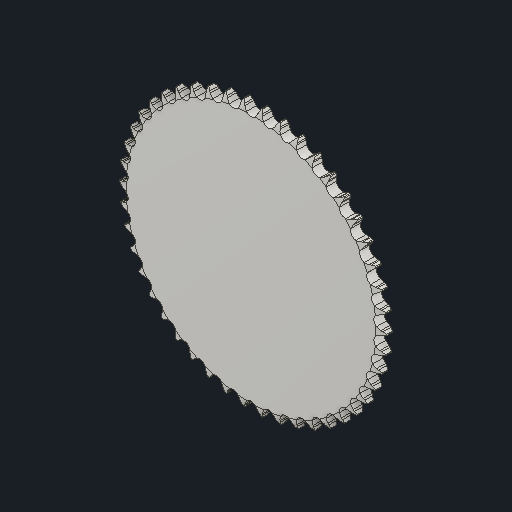
# Autodesk Inventor part: Roller Chain Sprocket2
Saved by Autodesk Inventor 2027 (Build 310192000, 192)
## iProperties
CustomPartVersion: 1
Created: 2026-06-06
Part Number: Roller Chain Sprocket2
Material: Steel
Document SubType Name: Modeling
Designer: W Ahmad
Density: 1 g/cm^3
Appearance: Steel
Author: W Ahmad
Autodesk Inventor part; units mm, degrees
ref_plane "YZ Plane" through (0, 0, 0) normal (1, 0, 0) x (0, 1, 0)
ref_plane "XZ Plane" through (0, 0, 0) normal (0, 1, 0) x (-1, 0, 0)
sketch "Theoretical Tooth Profile" plane through (0, 0, 0) normal (0, 0, 1) x (1, 0, 0)
  circle A0 centre (0, 0) radius 116.3133 construction
  line L0 (0, 0) -> (0, 116.3133) construction
  line L1 (0, 0) -> (15.838, 115.2299) construction
  circle A1 centre (0, 0) radius 120.8046
  arc A2 (-4.1451, 113.268) -> (4.1451, 113.268) centre (0, 116.3133) ccw
  line L2 (0, 116.3133) -> (15.838, 115.2299) construction
  line L3 (0, 116.3133) -> (6.5502, 121.1257) construction
  line L4 (6.5502, 121.1257) -> (-5.9584, 116.6908) construction
  arc A3 (7.8437, 120.5497) -> (6.453, 118.086) centre (14.1908, 115.3426) ccw
  arc A4 (-6.453, 118.086) -> (-7.8437, 120.5497) centre (-14.1908, 115.3426) ccw
  line L5 (-14.1908, 115.3426) -> (-6.453, 118.086) construction
  arc A5 (-5.9584, 116.6908) -> (-4.1451, 113.268) centre (6.5502, 121.1257) ccw
  line L6 (-5.9584, 116.6908) -> (-6.453, 118.086)
  arc A6 (4.1451, 113.268) -> (5.9584, 116.6908) centre (-6.5502, 121.1257) ccw
  line L7 (6.453, 118.086) -> (5.9584, 116.6908)
  line L8 (0, 0) -> (8.244, 120.523) construction
  point P0 (7.919, 115.7716)
  dimension "d0" = 232.6266
  dimension "d2" = 7.826
  dimension "d3" = 5.1435
  dimension "d10" = 126.304
  dimension "d11" = 16.783
  dimension "d12" = 8.128
  dimension "d13" = 13.2715
  dimension "d14" = 14.224
  dimension "d23" = 4.7625
  constraints: 18 end point, 15 point on circle, 7 centre point, 3 coincident, 3 point on line, 3 symmetric about line, 3 tangent, 1 equal radius, 1 midpoint, 1 parallel, 1 vertical, 1 other
  measures "d0" diameter of A0
  measures "d2" angle of L1 L0
  measures "d3" radius of A2
  measures "d10" angle of L3 L0
  measures "d11" angle of L4 L3
  measures "d12" distance of L2.start L3.end
  measures "d13" distance of L3.end L4.end
  measures "d14" distance of A3.centre L0.end
  measures "d23" distance from line of L8.end L2
sketch "Tooth Profile" plane through (0, 0, 0) normal (0, 0, 1) x (1, 0, 0)
  circle A0 centre (0, 0) radius 120.8046 projected
  line L0 (0, 0) -> (0, 116.3133) construction
  line L1 (0, 116.3133) -> (4.8026, 114.4719) construction
  arc A1 (-4.8026, 114.4719) -> (4.8026, 114.4719) centre (0, 116.3133) ccw
  line L2 (-4.8026, 114.4719) -> (0, 116.3133) construction
  arc A2 (-4.8026, 114.4719) -> (-7.5494, 120.5685) centre (-59.4451, 93.5203) ccw
  arc A3 (7.5494, 120.5685) -> (4.8026, 114.4719) centre (59.4451, 93.5203) ccw
  dimension "d44" = 138.043
  dimension "d45" = 5.1435
  dimension "d46" = 58.5216
  constraints: 8 point on circle, 7 end point, 3 centre point, 2 tangent, 1 coincident, 1 equal radius, 1 symmetric about line, 1 vertical
  measures "d44" angle of L1 L2
  measures "d45" radius of A1
  measures "d46" radius of A3
sketch "Section Profile" plane through (0, 0, 0) normal (1, 0, 0) x (0, 1, 0)
  line L0 (120.8046, 0) -> (-120.8046, 0) projected
  line L1 (107.0886, 4.5053) -> (-107.0886, 4.5053)
  line L2 (-107.0886, 4.5053) -> (-107.0886, -4.5053)
  line L3 (-107.0886, -4.5053) -> (107.0886, -4.5053)
  line L4 (107.0886, -4.5053) -> (107.0886, 4.5053)
  line L5 (107.0886, 4.5053) -> (120.8046, 4.5053) construction
  line L6 (120.8046, 4.5053) -> (120.8046, -4.5053) construction
  line L7 (120.8046, -4.5053) -> (107.0886, -4.5053) construction
  line L8 (107.0886, -4.5053) -> (107.0886, 4.5053)
  arc A0 (120.8046, 2.521) -> (112.8652, 4.5053) centre (112.8652, -12.3698) ccw
  arc A1 (112.8652, -4.5053) -> (120.8046, -2.521) centre (112.8652, 12.3698) ccw
  line L9 (112.8652, 4.5053) -> (0, 4.5053)
  line L10 (0, 4.5053) -> (0, -4.5053)
  line L11 (0, -4.5053) -> (112.8652, -4.5053)
  line L12 (0, 4.5053) -> (0, -4.5053)
  line L13 (120.8046, 2.521) -> (120.8046, -2.521)
  point P0 (0, 0)
  point P1 (0, 0)
  dimension "d30" = 9.0107
  dimension "d31" = 214.1773
  dimension "d32" = 9.0107
  dimension "d33" = 1.9844
  dimension "d34" = 16.8751
  dimension "d43" = 4.5053
  constraints: 26 end point, 7 midpoint, 5 perpendicular, 4 parallel, 4 point on circle, 3 point on line, 3 symmetric about line, 2 centre point, 2 horizontal, 2 tangent, 1 collinear, 1 other
  measures "d30" distance between parallel lines of L7 L5
  measures "d31" distance between parallel lines of L2 L4
  measures "d32" distance between parallel lines of L3 L1
  measures "d33" distance from line of L13.start L5
  measures "d34" radius of A0
  measures "d43" distance between parallel lines of L3 L0
revolve "Shroud" add sketch "Section Profile" angle 360 about axis through (0, 0, 4.5053) along (0, 0, -1) contours L10 L3 L2 L0 | L0 L2 L1 L10
revolve "Strand" add sketch "Section Profile" angle 360 about axis through (0, 0, 4.5053) along (0, 0, -1) contours L13 A1 L11 L4 L0 | L0 L4 L9 A0 L13 | L4 L3 L10 L0 | L0 L10 L1 L4
fillet "Fillet2" [suppressed]
pattern_of_one "Strand Pattern"
extrude "Theoretical Tooth" cut sketch "Theoretical Tooth Profile" along normal through all both and the other way through all contours A3 L7 A6 A2 A5 L6 A4 A1 picked at (0.8721, 115.7708)
extrude "Tooth" [suppressed]
pattern_circular "Tooth Pattern" count 46 over 360 about axis through (0, 0, -10) along (0, 0, 1) of "Theoretical Tooth"
ref_plane "Timing Plane" through (0, 116.3133, 0) normal (1, 0, 0) x (0, 1, 0)
equation "\"d3\" = 0.5 * da_Dr + da_SC"
equation "\"d12\" = 0.8 * da_Dr"
equation "\"d13\" = 1.3 * da_Dr + da_SC"
equation "\"d14\" = 1.4 * da_Dr"
equation "\"d23\" = da_Ha"
equation "\"d44\" = da_Alfa"
equation "\"d45\" = da_Ri"
equation "\"d46\" = da_Re"
equation "\"d30\" = da_Bf"
equation "\"d31\" = da_Ds"
equation "\"d32\" = da_Bs"
equation "\"d33\" = da_Ba"
equation "\"d34\" = da_Rx"
equation "\"d51\" = da_Ra"
equation "\"d40\" = da_pt"
equation "\"form_type\" = 0"
equation "\"da_p\" = 15.875"
equation "\"da_Dr\" = 10.16"
equation "\"da_SC\" = 0.0635"
equation "\"da_Ha\" = 4.7625"
equation "\"da_pt\" = 18.1102"
equation "\"da_Bf\" = 9.01065"
equation "\"da_Ba\" = 1.98438"
equation "\"da_Rx\" = 16.87513"
equation "\"da_Ra\" = 0.635"
equation "\"da_Bs\" = 9.01065"
equation "\"da_Ds\" = 214.17728"
equation "\"da_Re\" = 58.5216"
equation "\"da_Ri\" = 5.1435"
equation "\"da_Alfa\" = 138.043deg"
body "Solid1"
